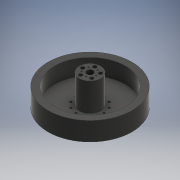
# Autodesk Inventor part: SG02
Saved by Autodesk Inventor 2017 (Build 210142000, 142)
## iProperties
Created: 2019-09-21
Part Number: SG02
Material: ABS Plastic
Document SubType Name: Modeling
Designer: Dell
Density: 1.06 g/cm^3
Appearance: Smooth - Black
Author: Dell
Autodesk Inventor part; units mm, degrees
ref_plane "YZ Plane" through (0, 0, 0) normal (1, 0, 0) x (0, 1, 0)
ref_plane "XZ Plane" through (0, 0, 0) normal (0, 1, 0) x (-1, 0, 0)
ref_plane "XY Plane" through (0, 0, 0) normal (0, 0, 1) x (1, 0, 0)
sketch "Sketch2" plane through (0, 0, 0) normal (0, 0, 1) x (1, 0, 0)
  circle A0 centre (0, 0) radius 45
  dimension "d0" = 90
  constraints: 1 centre point, 1 coincident
  measures "d0" diameter of A0
extrude "Extrusion1" add sketch "Sketch2" along normal blind 10
sketch "Sketch4" plane through (0, 0, 10) normal (0, 0, 1) x (1, 0, 0)
  circle A0 centre (0, 0) radius 11.5
  dimension "d14" = 23
  constraints: 1 centre point, 1 coincident
  measures "d14" diameter of A0
extrude "Extrusion3" add sketch "Sketch4" along normal blind 23
sketch "Sketch5" plane through (0, 0, 33) normal (0, 0, 1) x (1, 0, 0)
  circle A0 centre (-8, 0) radius 2
  circle A1 centre (0, 0) radius 3.5
  circle A2 centre (0, 0) radius 11.5 construction
  circle A3 centre (-2.4721, -7.6085) radius 2
  circle A4 centre (6.4721, -4.7023) radius 2
  circle A5 centre (6.4721, 4.7023) radius 2
  circle A6 centre (-2.4721, 7.6085) radius 2
  dimension "d19" = 4
  dimension "d20" = 8
  dimension "d21" = 360
  dimension "d22" = 7
  constraints: 7 centre point, 1 coincident, 1 horizontal alignment, 11 other
  measures "d19" diameter of A0
  measures "d20" distance of point (0, 0) A0.centre
  measures "d22" diameter of A1
extrude "Extrusion4" cut sketch "Sketch5" against normal through all
sketch "Sketch8" plane through (0, 0, 33) normal (0, 0, 1) x (1, 0, 0)
  circle A0 centre (2.0086, 6.1819) radius 0.75
  circle A1 centre (-5.2586, 3.8206) radius 0.75
  circle A2 centre (-5.2586, -3.8206) radius 0.75
  circle A3 centre (2.0086, -6.1819) radius 0.75
  circle A4 centre (6.5, 0) radius 0.75
  circle A5 centre (-2.4721, 7.6085) radius 2 construction
  circle A6 centre (6.4721, 4.7023) radius 2 construction
  circle A7 centre (-2.4721, 7.6085) radius 2 projected
  line L0 (6.4721, 4.7023) -> (-2.4721, 7.6085) construction
  line L1 (0, 0) -> (2.0086, 6.1819) construction
  point P0 (2, 6.1554)
  dimension "d44" = 1.5
  dimension "d45" = 6.5
  dimension "d48" = 360
  constraints: 5 centre point, 4 end point, 1 midpoint, 1 point on line, 11 other
  measures "d44" diameter of A0
  measures "d45" distance of L1.start L1.end
extrude "Extrusion7" cut sketch "Sketch8" against normal through all contours A0 | A1 | A2 | A3 | A4
sketch "Sketch9" plane through (0, 0, 10) normal (0, 0, 1) x (1, 0, 0)
  circle A0 centre (0, 0) radius 22
  circle A1 centre (0, 0) radius 38
  dimension "d52" = 44
  dimension "d53" = 76
  constraints: 2 centre point, 2 coincident
  measures "d52" diameter of A0
  measures "d53" diameter of A1
extrude "Extrusion8" cut sketch "Sketch9" against normal blind 7.35
sketch "Sketch10" plane through (0, 0, 0) normal (0, 0, -1) x (-1, 0, 0)
  circle A0 centre (0, 0) radius 22 construction
  circle A1 centre (0, 0) radius 38 construction
  circle A2 centre (0, 0) radius 22 construction
  circle A3 centre (0, 0) radius 38 construction
  circle A4 centre (15, 0) radius 1.25
  circle A5 centre (12.9904, 7.5) radius 1.25
  circle A6 centre (7.5, 12.9904) radius 1.25
  circle A7 centre (0, 15) radius 1.25
  circle A8 centre (-7.5, 12.9904) radius 1.25
  circle A9 centre (-12.9904, 7.5) radius 1.25
  circle A10 centre (-15, 0) radius 1.25
  circle A11 centre (-12.9904, -7.5) radius 1.25
  circle A12 centre (-7.5, -12.9904) radius 1.25
  circle A13 centre (0, -15) radius 1.25
  circle A14 centre (7.5, -12.9904) radius 1.25
  circle A15 centre (12.9904, -7.5) radius 1.25
  dimension "d56" = 2.5
  dimension "d59" = 360
  dimension "d66" = 15
  constraints: 14 centre point, 1 coincident, 1 horizontal alignment, 25 other
  measures "d56" diameter of A4
  measures "d66" distance of point (0, 0) A4.centre
extrude "Extrusion9" cut sketch "Sketch10" against normal through all
sketch "Sketch13" plane through (0, 0, 10) normal (0, 0, 1) x (1, 0, 0)
  circle A0 centre (0, 0) radius 45 projected
  circle A1 centre (0, 0) radius 38 projected
extrude "Extrusion10" add sketch "Sketch13" along normal blind 10
sketch "Sketch14" plane through (0, 0, 2.65) normal (0, 0, 1) x (1, 0, 0)
  circle A0 centre (0, 0) radius 22 projected
  circle A1 centre (0, 0) radius 11.5 projected
extrude "Extrusion11" cut sketch "Sketch14" along normal up to surface (7.35 mm away) from surface at 0
body "Solid1"
